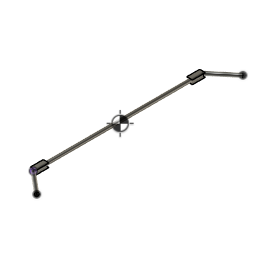
Maya Wing Attach Comp. Test v16 (Autodesk Fusion 360 design; units mm, degrees)
Autodesk Fusion 360 part; units mm, degrees
sketch "Sketch1" plane through (0, 0, 0) normal (0, 1, 0) x (1, 0, 0)
  circle A0 centre (0, 0) radius 7.9375
  circle A1 centre (0, 0) radius 7.0485
  line L0 (-12.7, 7.9375) -> (12.7, 7.9375)
  line L1 (12.7, -7.9375) -> (-12.7, -7.9375)
  line L2 (12.7, -7.9375) -> (12.7, -9.525)
  line L3 (12.7, -9.525) -> (-12.7, -9.525)
  line L4 (-12.7, -7.9375) -> (-12.7, -9.525)
  line L5 (12.7, 7.9375) -> (12.7, 9.525)
  line L6 (12.7, 9.525) -> (-12.7, 9.525)
  line L7 (-12.7, 9.525) -> (-12.7, 7.9375)
  line L8 (12.7, -7.9375) -> (12.7, 7.9375) construction
  point P0 (0, -7.9375)
  dimension "d1" = 15.875
  dimension "d2" = 0.889
  dimension "d9" = 1.5875
  dimension "d10" = 25.4
  constraint coincident A0.centre A1.centre
  constraint tangent A0 L0
  constraint horizontal L0
  constraint horizontal L1
  constraint tangent A0 L1
  constraint perpendicular L1 L2
  constraint perpendicular L2 L3
  constraint perpendicular L3 L4
  constraint perpendicular L0 L5
  constraint perpendicular L5 L6
  constraint perpendicular L6 L7
  constraint equal L2 L5
  constraint equal L0 L3
  constraint vertical L8
  constraint coincident L1 P0
  constraint coincident A0 P0
  constraint midpoint L1 P0
  measures "d1" diameter of A0
  measures "d2" distance of A0 A1
  measures "d9" distance of L0.end L5.end
  measures "d10" distance of L5.end L6.end
extrude "Extrude7" add sketch "Sketch1" along normal blind 57.15 contours L1 L2 L3 L4 | L0 L5 L6 L7 makes body 1 at (4.2333, 19.05, 9.525) makes body 2 at (4.2333, 19.05, -9.525)
sketch "Pipes" plane through (0, 0, 0) normal (0, 0, 1) x (1, 0, 0)
  line L0 (0, 0) -> (0, 749.3)
  line L1 (0, 749.3) -> (97.2876, 830.934)
  line L2 (0, 0) -> (97.2876, -81.634)
  dimension "d31" = 130
  dimension "d32" = 130
  dimension "d33" = 749.3
  dimension "d34" = 127
  constraint coincident L0.start L2.start
  constraint vertical L0
  constraint equal L1 L2
  measures "d31" angle of L0 L2
  measures "d32" angle of L0 L1
  measures "d33" distance of L0.start L0.end
  measures "d34" distance of L0.end L1.end
ref_plane "WorkPlane1" through (0, 749.3, 0) normal (0, 1, 0) x (0, 0, 1)
sketch "Sketch6" plane through (0, 749.3, 0) normal (0, 1, 0) x (1, 0, 0)
  line L0 (-12.7, 9.525) -> (-12.7, 7.9375)
  line L1 (-12.7, 7.9375) -> (12.7, 7.9375)
  line L2 (12.7, 7.9375) -> (12.7, 9.525)
  line L3 (12.7, 9.525) -> (-12.7, 9.525)
  line L4 (12.7, -7.9375) -> (-12.7, -7.9375)
  line L5 (-12.7, -7.9375) -> (-12.7, -9.525)
  line L6 (-12.7, -9.525) -> (12.7, -9.525)
  line L7 (12.7, -9.525) -> (12.7, -7.9375)
extrude "Extrude8" add sketch "Sketch6" against normal blind 57.15 separate body makes body 3 at (-4.2333, 730.25, 9.525) makes body 4 at (4.2333, 730.25, -9.525)
sketch "Sketch7" plane through (0, 0, 0) normal (0, 1, 0) x (1, 0, 0)
pipe "Pipe3" add diameter 15.875 wall 0.889 path "Pipes" along L2 L0 L1 separate body makes body 5
sketch "Sketch8" plane through (0, 0, -7.9375) normal (0, 0, 1) x (-1, 0, 0)
  line L0 (12.7, 0) -> (-12.7, 0)
  line L1 (-12.7, 0) -> (-12.7, -57.15)
  line L2 (-12.7, -57.15) -> (12.7, -57.15)
  line L3 (12.7, -57.15) -> (12.7, 0)
  line L4 (8.7917, -7.9039, 2.7263) -> (12.7, 0, 15.875)
  point P0 (12.7, 0)
  constraint coincident P0 L0.start
equation "d9 = ( 1 / 16 ) * 1 in"
named bodies: "Pipes"
